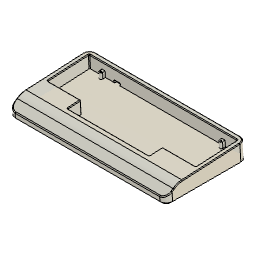
SK-Vault35 Ultra HHKB (Autodesk Fusion 360 design; units mm, degrees)
Autodesk Fusion 360 part; units mm, degrees
sketch "Base Plane Sketch" plane through (0, 0, 0) normal (0, 0, 1) x (1, 0, 0)
  line L0 (0, 0) -> (209.55, 0) construction
  line L1 (209.55, 0) -> (209.55, -57.15) construction
  line L2 (209.55, -57.15) -> (161.925, -57.15) construction
  line L3 (161.925, -57.15) -> (161.925, -76.2) construction
  line L4 (0, 0) -> (0, -57.15) construction
  line L5 (0, -57.15) -> (47.625, -57.15) construction
  line L6 (47.625, -57.15) -> (47.625, -76.2) construction
  line L7 (47.625, -76.2) -> (161.925, -76.2) construction
  line L8 (-7.5, 7.5) -> (217.05, 7.5)
  line L9 (217.05, 7.5) -> (217.05, -64.65)
  line L10 (217.05, -64.65) -> (169.425, -64.65)
  line L11 (169.425, -64.65) -> (169.425, -83.7)
  line L12 (40.125, -83.7) -> (169.425, -83.7)
  line L13 (40.125, -64.65) -> (40.125, -83.7)
  line L14 (-7.5, -64.65) -> (40.125, -64.65)
  line L15 (-7.5, 7.5) -> (-7.5, -64.65)
  line L16 (-7.5, -64.65) -> (-7.5, -83.7)
  line L17 (-7.5, -83.7) -> (40.125, -83.7)
  line L18 (169.425, -83.7) -> (217.05, -83.7)
  line L19 (217.05, -83.7) -> (217.05, -64.65)
  line L20 (-7.5, -83.7) -> (-7.5, -90.7)
  line L21 (-7.5, -90.7) -> (217.05, -90.7)
  line L22 (217.05, -90.7) -> (217.05, -83.7)
  line L23 (0, 0) -> (19.05, 0) construction
  line L24 (19.05, 0) -> (19.05, -19.05) construction
  line L25 (19.05, -19.05) -> (0, -19.05) construction
  line L26 (0, -19.05) -> (0, 0) construction
  line L27 (0, -19.05) -> (19.05, 0) construction
  line L28 (19.05, -19.05) -> (0, 0) construction
  line L29 (16.525, -2.525) -> (2.525, -2.525) construction
  line L30 (2.525, -2.525) -> (2.525, -16.525) construction
  line L31 (2.525, -16.525) -> (16.525, -16.525) construction
  line L32 (16.525, -16.525) -> (16.525, -2.525) construction
  line L33 (16.525, -2.525) -> (2.525, -16.525) construction
  line L34 (2.525, -2.525) -> (16.525, -16.525) construction
  line L35 (9.525, -2.525) -> (9.525, 0.575) construction
  line L36 (0, -57.15) -> (19.05, -57.15) construction
  line L37 (19.05, -57.15) -> (19.05, -38.1) construction
  line L38 (19.05, -38.1) -> (0, -38.1) construction
  line L39 (0, -38.1) -> (0, -57.15) construction
  line L40 (0, -57.15) -> (19.05, -38.1) construction
  line L41 (0, -38.1) -> (19.05, -57.15) construction
  line L42 (16.525, -40.625) -> (2.525, -40.625) construction
  line L43 (2.525, -40.625) -> (2.525, -54.625) construction
  line L44 (2.525, -54.625) -> (16.525, -54.625) construction
  line L45 (16.525, -54.625) -> (16.525, -40.625) construction
  line L46 (16.525, -40.625) -> (2.525, -54.625) construction
  line L47 (2.525, -40.625) -> (16.525, -54.625) construction
  line L48 (9.525, -54.625) -> (9.525, -57.725) construction
  circle A0 centre (2.266, -54.884) radius 2.25
  line L49 (-1.075, 1.075) -> (-1.075, -57.15)
  line L50 (0, -58.225) -> (46.55, -58.225)
  line L51 (46.55, -58.225) -> (46.55, -77.275)
  line L52 (46.55, -77.275) -> (163, -77.275)
  line L53 (163, -58.225) -> (163, -77.275)
  line L54 (210.625, -58.225) -> (163, -58.225)
  line L55 (210.625, 1.075) -> (210.625, -58.225)
  line L56 (0, 1.075) -> (210.625, 1.075)
  line L57 (-1.075, -57.15) -> (-1.075, -58.225)
  line L58 (-1.075, -58.225) -> (0, -58.225)
  line L59 (0, 1.075) -> (-1.075, 1.075)
  line L60 (209.55, 0) -> (190.5, 0) construction
  line L61 (190.5, 0) -> (190.5, -19.05) construction
  line L62 (190.5, -19.05) -> (209.55, -19.05) construction
  line L63 (209.55, -19.05) -> (209.55, 0) construction
  circle A1 centre (207.284, -54.884) radius 2.25
  line L64 (190.5, -9.525) -> (209.55, -9.525) construction
  line L65 (200.025, -19.05) -> (200.025, 0) construction
  circle A2 centre (19.05, -2.525) radius 2.25
  line L66 (19.05, -2.525) -> (190.5, -2.525) construction
  circle A3 centre (190.5, -2.525) radius 2.25
  line L67 (21.3, -2.525) -> (21.3, 1.075)
  line L68 (4.516, -54.884) -> (4.516, -58.225)
  line L69 (2.266, -52.634) -> (-1.075, -52.634)
  line L70 (205.034, -54.884) -> (205.034, -58.225)
  line L71 (207.284, -52.634) -> (210.625, -52.634)
  line L72 (192.75, -2.525) -> (192.75, 1.075)
  line L73 (188.25, -2.525) -> (188.25, 1.075)
  line L74 (16.8193, -2.2307) -> (16.8193, 1.075)
  point P0 (9.525, -9.525)
  point P1 (9.525, -47.625)
  dimension "d1" = 209.55
  dimension "d2" = 57.15
  dimension "d3" = 47.625
  dimension "d4" = 19.05
  dimension "d5" = 57.15
  dimension "d6" = 47.625
  dimension "d7" = 19.05
  dimension "d9" = 7.5
  dimension "d39" = 7
  dimension "d98" = 19.05
  dimension "d99" = 19.05
  dimension "d100" = 14
  dimension "d101" = 14
  dimension "d102" = 3.1
  dimension "d103" = 19.05
  dimension "d104" = 19.05
  dimension "d105" = 14
  dimension "d106" = 14
  dimension "d108" = 3.1
  dimension "d114" = 1.075
  dimension "d115" = 45.359
  dimension "d116" = 7.259
  dimension "d117" = 19.05
  dimension "d118" = 19.05
  dimension "d120" = 45.359
  dimension "d121" = 7.259
  dimension "d122" = 4.5
  dimension "d123" = 19.05
  constraint coincident L0.start L4.start
  constraint horizontal L0
  constraint perpendicular L0 L1
  constraint perpendicular L1 L2
  constraint perpendicular L2 L3
  constraint perpendicular L0 L4
  constraint perpendicular L4 L5
  constraint perpendicular L5 L6
  constraint perpendicular L12 L16
  constraint perpendicular L13 L17
  constraint perpendicular L9 L18
  constraint perpendicular L10 L19
  constraint vertical L20
  constraint perpendicular L19 L21
  constraint perpendicular L18 L22
  constraint horizontal L23
  constraint vertical L24
  constraint horizontal L25
  constraint vertical L26
  constraint horizontal L29
  constraint perpendicular L29 L30
  constraint parallel L29 L31
  constraint parallel L30 L32
  constraint coincident L33 P0
  constraint coincident L34 P0
  constraint midpoint L27 P0
  constraint midpoint L29 L35.start
  constraint horizontal L36
  constraint vertical L37
  constraint horizontal L38
  constraint vertical L39
  constraint horizontal L42
  constraint perpendicular L42 L43
  constraint parallel L42 L44
  constraint parallel L43 L45
  constraint coincident L46 P1
  constraint coincident L47 P1
  constraint midpoint L40 P1
  constraint midpoint L44 L48.start
  constraint perpendicular L50 L57
  constraint perpendicular L57 L58
  constraint perpendicular L49 L59
  constraint horizontal L60
  constraint vertical L61
  constraint horizontal L62
  constraint vertical L63
  constraint midpoint L61 L64.start
  constraint midpoint L63 L64.end
  constraint midpoint L62 L65.start
  constraint midpoint L60 L65.end
  constraint coincident A2.centre L66.start
  constraint coincident L61 L66.end
  constraint perpendicular L61 L66
  constraint coincident L66.end A3.centre
  constraint coincident A2 L67.start
  constraint coincident L66 L67.start
  constraint coincident L56 L67.end
  constraint tangent A2 L67
  constraint coincident A0 L68.start
  constraint coincident L50 L68.end
  constraint tangent A0 L68
  constraint perpendicular L50 L68
  constraint coincident A0 L69.start
  constraint coincident L49 L69.end
  constraint tangent A0 L69
  constraint perpendicular L49 L69
  constraint coincident A1 L70.start
  constraint coincident L54 L70.end
  constraint tangent A1 L70
  constraint perpendicular L54 L70
  constraint coincident A1 L71.start
  constraint coincident L55 L71.end
  constraint tangent A1 L71
  constraint perpendicular L55 L71
  constraint coincident A3 L72.start
  constraint coincident L56 L72.end
  constraint tangent A3 L72
  constraint perpendicular L56 L72
  constraint coincident L66 L73.start
  constraint coincident A3 L73.start
  constraint coincident L56 L73.end
  constraint tangent A3 L73
  constraint coincident L27 L74.start
  constraint coincident A2 L74.start
  constraint coincident L56 L74.end
  constraint perpendicular L56 L74
  constraint equal A0 A2
  constraint equal A1 A2
  constraint equal A2 A3
  measures "d1" distance of L0.start L0.end
  measures "d2" distance of L0.end L1.end
  measures "d3" distance of L1.end L2.end
  measures "d4" distance of L2.end L3.end
  measures "d5" distance of L0.start L4.end
  measures "d6" distance of L4.end L5.end
  measures "d7" distance of L5.end L6.end
  measures "d39" distance of L16.end L20.end
  measures "d98" distance of L0.start L23.end
  measures "d99" distance of L0.start L25.end
  measures "d100" distance of L30.end L31.end
  measures "d101" distance of L29.end L30.end
  measures "d102" distance of L35.start L35.end
  measures "d103" distance of L4.end L36.end
  measures "d104" distance of L4.end L38.end
  measures "d105" distance of L43.end L44.end
  measures "d106" distance of L42.end L43.end
  measures "d108" distance of L48.start L48.end
  measures "d115" vertical distance of P0 A0.centre
  measures "d116" horizontal distance of P0 A0.centre
  measures "d117" distance of L0.end L60.end
  measures "d118" distance of L0.end L62.end
  measures "d120" distance of A1.centre L64
  measures "d121" distance of A1.centre L65
  measures "d122" diameter of A2
  measures "d123" distance of L4 A2.centre
extrude "External Base Extrude" add sketch "Base Plane Sketch" along normal blind 21.06
extrude "Internal Base Extrude" add sketch "Base Plane Sketch" 1 faces at (195.028, -73.0667, 0) along normal blind 3 contours A0 | A0 L49 L50 L57 L58 L68 L69 | A0 L49 L50 L51 L52 L53 L54 L55 L56 L59 A1 A2 A3 L67 L68 L69 L70 L71 L72 L73 L74 | L56 A2 L67 L74 | A2 | L54 L55 A1 L70 L71 | L56 A3 L72 L73 | A1 | A3
sketch "Side Plane Sketch" plane through (-7.5, 0, 0) normal (-1, 0, 0) x (0, -1, 0)
  line L0 (90.7, 0) -> (90.7, 21.06)
  line L1 (90.7, 21.06) -> (-7.5, 21.06)
  line L2 (-7.5, 21.06) -> (-7.5, 0)
  line L3 (-7.5, 0) -> (90.7, 0)
  line L4 (90.7, 21.06) -> (107.8598, 10)
  line L5 (107.8598, 10) -> (107.8598, 0)
  line L6 (107.8598, 0) -> (90.7, 0)
  dimension "d149" = 10
  constraint coincident L0.end L1.start
  constraint perpendicular L3 L5
  constraint coincident L0.start L3.end
  constraint perpendicular L0 L6
  measures "d149" distance of L4.end L5.end
extrude "Wrist Wrest Extrude" add sketch "Side Plane Sketch" against normal up to surface (224.55 mm away) contours L0 L4 L5 L6
fillet "Outside Vertical Fillets" radius 9 4 edges at (-7.5, -107.8598, 5) (217.05, -107.8598, 5) (217.05, 7.5, 10.53) (-7.5, 7.5, 10.53)
fillet "Wrist Wrest Angle Fillet" radius 23.5 1 edges at (104.775, -90.7, 21.06)
fillet "Inside Case Vertical Fillets" radius 1 8 edges at (210.625, 1.075, 12.03) (-1.075, 1.075, 12.03) (-1.075, -58.225, 12.03) (46.55, -58.225, 12.03) (46.55, -77.275, 12.03) (163, -77.275, 12.03) (163, -58.225, 12.03) (210.625, -58.225, 12.03)
chamfer "Top Outside Edge Chamfer" distance 1 angle 45 12 edges at (-7.5, -42.6415, 21.06) (-7.5, -90.4185, 20.1037) (-7.5, -97.6869, 16.5567) (-4.864, -105.2238, 11.699) (104.775, -107.8598, 10) (214.414, -105.2238, 11.699) (217.05, -97.6869, 16.5567) (217.05, -90.4185, 20.1037) (217.05, -42.6415, 21.06) (214.414, 4.864, 21.06) (104.775, 7.5, 21.06) (-4.864, 4.864, 21.06)
chamfer "Top Inside Edge Chamfer" distance 1 angle 45 16 edges at (104.775, 1.075, 21.06) (210.3321, 0.7821, 21.06) (210.625, -28.575, 21.06) (210.3321, -57.9321, 21.06) (186.8125, -58.225, 21.06) (163.2929, -58.5179, 21.06) (163, -67.75, 21.06) (162.7071, -76.9821, 21.06) (104.775, -77.275, 21.06) (46.8429, -76.9821, 21.06) (46.55, -67.75, 21.06) (46.2571, -58.5179, 21.06) (22.7375, -58.225, 21.06) (-0.7821, -57.9321, 21.06) (-1.075, -28.575, 21.06) (-0.7821, 0.7821, 21.06)
sketch "USB C Hole Internal" plane through (0, 1.075, 0) normal (0, -1, 0) x (1, 0, 0)
  line L0 (193, 10.9) -> (193, 3)
  line L1 (193, 3) -> (209.05, 3)
  line L2 (209.05, 3) -> (209.05, 17.06)
  line L3 (209.05, 17.06) -> (0.5, 17.06)
  line L4 (0.5, 17.06) -> (0.5, 3)
  line L5 (0.5, 3) -> (16.55, 3)
  line L6 (16.55, 3) -> (16.55, 10.9)
  line L7 (16.55, 10.9) -> (21.55, 10.9)
  line L8 (21.55, 10.9) -> (21.55, 3)
  line L9 (21.55, 3) -> (188, 3)
  line L10 (188, 3) -> (188, 10.9)
  line L11 (188, 10.9) -> (193, 10.9)
  line L12 (0.5, 3) -> (0, 3) construction
  line L13 (34.925, 3) -> (38.1, 3) construction
  line L14 (41.275, 6.66) -> (34.925, 6.66)
  line L15 (33.375, 5.11) -> (33.375, 4.55)
  line L16 (33.375, 3) -> (41.275, 3)
  line L17 (42.825, 4.55) -> (42.825, 5.11)
  line L18 (42.825, 6.66) -> (33.375, 3) construction
  line L19 (33.375, 6.66) -> (42.825, 3) construction
  arc A0 (34.925, 6.66) -> (33.375, 5.11) centre (34.925, 5.11) ccw
  arc A1 (42.825, 5.11) -> (41.275, 6.66) centre (41.275, 5.11) ccw
  arc A2 (41.275, 3) -> (42.825, 4.55) centre (41.275, 4.55) ccw
  arc A3 (33.375, 4.55) -> (34.925, 3) centre (34.925, 4.55) ccw
  line L20 (209.625, 20.06) -> (-0.075, 20.06)
  line L21 (-0.075, 20.06) -> (-0.075, 3)
  line L22 (-0.075, 3) -> (209.625, 3)
  line L23 (209.625, 3) -> (209.625, 20.06)
  point P0 (38.1, 4.83)
  dimension "d75" = 0.5
  dimension "d79" = 1.55
  dimension "d80" = 9.45
  dimension "d82" = 38.1
  dimension "d83" = 3.66
  constraint coincident L4.end L5.start
  constraint perpendicular L4 L12
  constraint parallel L5 L13
  constraint horizontal L14
  constraint perpendicular L14 L15
  constraint parallel L14 L16
  constraint parallel L15 L17
  constraint coincident L18 P0
  constraint coincident L19 P0
  constraint coincident L19.start L15
  constraint coincident L19.start L14
  constraint tangent L15 A0
  constraint tangent L14 A0
  constraint coincident L18.start L14
  constraint coincident L18.start L17
  constraint tangent L14 A1
  constraint tangent L17 A1
  constraint equal A0 A1
  constraint coincident L19.end L17
  constraint coincident L19.end L16
  constraint tangent L17 A2
  constraint tangent L16 A2
  constraint equal A0 A2
  constraint coincident L12.end L13
  constraint coincident L16.start L15
  constraint tangent L13 A3
  constraint tangent L15 A3
  constraint equal A0 A3
  measures "d75" distance of L4.end L12.end
  measures "d79" radius of A0
  measures "d80" distance of L15 L17
  measures "d82" distance of L12.end L13.end
  measures "d83" distance of L13.end L14
extrude "Internal USB C Extrude Cut" cut sketch "USB C Hole Internal" against normal blind 24 contours L9 L14 L15 L16 L17 A0 A1 A2 A3 L22
sketch "USB C Hole External" plane through (0, 7.5, 0) normal (0, 1, 0) x (-1, 0, 0)
  arc A0 (-42.825, 4.55) -> (-41.275, 3) centre (-41.275, 4.55) ccw
  line L0 (-42.825, 4.55) -> (-42.825, 5.11)
  arc A1 (-41.275, 6.66) -> (-42.825, 5.11) centre (-41.275, 5.11) ccw
  line L1 (-41.275, 6.66) -> (-34.925, 6.66)
  arc A2 (-33.375, 5.11) -> (-34.925, 6.66) centre (-34.925, 5.11) ccw
  line L2 (-33.375, 5.11) -> (-33.375, 4.55)
  arc A3 (-34.925, 3) -> (-33.375, 4.55) centre (-34.925, 4.55) ccw
  line L3 (-42.825, 4.83) -> (-33.375, 4.83) construction
  line L4 (-38.1, 6.66) -> (-38.1, 3) construction
  line L5 (-34.925, 8.91) -> (-41.275, 8.91)
  line L6 (-45.075, 5.11) -> (-45.075, 4.55)
  line L7 (-41.275, 0.75) -> (-34.925, 0.75)
  line L8 (-31.125, 4.55) -> (-31.125, 5.11)
  line L9 (-31.125, 8.91) -> (-45.075, 0.75) construction
  line L10 (-45.075, 8.91) -> (-31.125, 0.75) construction
  arc A4 (-41.275, 8.91) -> (-45.075, 5.11) centre (-41.275, 5.11) ccw
  arc A5 (-31.125, 5.11) -> (-34.925, 8.91) centre (-34.925, 5.11) ccw
  arc A6 (-34.925, 0.75) -> (-31.125, 4.55) centre (-34.925, 4.55) ccw
  arc A7 (-45.075, 4.55) -> (-41.275, 0.75) centre (-41.275, 4.55) ccw
  line L11 (-1.5, 0) -> (-1.5, 20.06)
  line L12 (-208.05, 20.06) -> (-208.05, 0)
  line L13 (-1.5, 20.06) -> (-208.05, 20.06)
  line L14 (-34.925, 3) -> (-41.275, 3)
  line L15 (-208.05, 0) -> (-1.5, 0)
  point P0 (-38.1, 4.83)
  dimension "d86" = 13.95
  dimension "d87" = 8.16
  dimension "d88" = 3.8
  constraint midpoint L0 L3.start
  constraint midpoint L2 L3.end
  constraint midpoint L1 L4.start
  constraint horizontal L5
  constraint perpendicular L5 L6
  constraint parallel L5 L7
  constraint parallel L6 L8
  constraint coincident L9 P0
  constraint coincident L10 P0
  constraint midpoint L3 P0
  constraint coincident L10.start L6
  constraint coincident L10.start L5
  constraint tangent L6 A4
  constraint tangent L5 A4
  constraint coincident L9.start L5
  constraint coincident L9.start L8
  constraint tangent L5 A5
  constraint tangent L8 A5
  constraint equal A4 A5
  constraint coincident L10.end L8
  constraint coincident L10.end L7
  constraint tangent L8 A6
  constraint tangent L7 A6
  constraint equal A4 A6
  constraint coincident L9.end L7
  constraint coincident L9.end L6
  constraint tangent L7 A7
  constraint tangent L6 A7
  constraint equal A4 A7
  measures "d86" distance of L9.end L10.end
  measures "d87" distance of L10.start L9.end
  measures "d88" radius of A4
extrude "External USB C Extrude Cut" cut sketch "USB C Hole External" against normal blind 4 contours A0 L0 A1 L1 A2 L2 A3 L14 | L5 L6 L7 L8 A4 A5 A6 A7
ref_plane "WorkPlane2" through (104.775, -107.8598, 0) normal (0, 0.052336, 0.99863) x (1, 0, 0)
extrude "Extrude18" add 1 faces at (70.35, -69.4065, 0) along direction (0, 0, -1) up to surface end surface through (104.775, -107.8598, 0) normal (0, 0.052336, 0.99863) offset 0
chamfer "Chamfer9" distance 3 angle 45 8 edges at (217.05, -50.1799, -3.0229) (214.414, -105.2238, -0.1381) (104.775, -107.8598, 0) (-4.864, -105.2238, -0.1381) (-7.5, -50.1799, -3.0229) (-4.864, 4.864, -5.9076) (104.775, 7.5, -6.0458) (214.414, 4.864, -5.9076)
extrude "Screw Post Extrude" add sketch "Base Plane Sketch" along normal blind 8.41 from surface at 3 contours A0 | A0 L49 L50 L57 L58 L68 L69 | L56 A2 L67 L74 | A2 | L54 L55 A1 L70 L71 | L56 A3 L72 L73 | A1 | A3
hole "Top Left Screw Hole" at (19.05, -2.525, 11.41) direction (0, 0, -1) diameter 1.8 depth 4 tip angle 180
hole "Top Right Screw Hole" at (190.5, -2.525, 11.41) direction (0, 0, -1) diameter 1.8 depth 4 tip angle 180
hole "Bottom Right Screw Hole" at (207.284, -54.884, 11.41) direction (0, 0, -1) diameter 1.8 depth 4 tip angle 180
hole "Bottom Left Screw Hole" at (2.266, -54.884, 11.41) direction (0, 0, -1) diameter 1.8 depth 4 tip angle 180
move_body "Rotate Case" bodies 1 to x (1, 0, 0) y (0, 0.99863, 0.052336) z (0, -0.052336, 0.99863) at (0, 0.0092, 5.6491)
equation "d3 = 19.05 mm * 2.5"
equation "d5 = 3 * 19.05 mm"
equation "d6 = 19.05 mm * 2.5"
equation "d10 = 18.06 mm + 3 mm"
equation "d114 = 0.575 mm + 0.5 mm"
equation "d130 = 7.9 mm + 0.51 mm"
